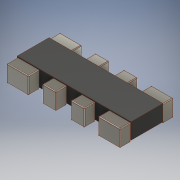
# Autodesk Inventor part: ResistorArray-1632
Saved by Autodesk Inventor 2018 (Build 220112000, 112)
## iProperties
Created: 2018-09-29
Part Number: ResistorArray-1632
Material: Copper
Document SubType Name: Modeling
Designer: Bradley
Density: 8.94 g/cm^3
Appearance: Copper - Satin
Author: Bradley
Autodesk Inventor part; units mm, degrees
ref_plane "YZ Plane" through (0, 0, 0) normal (1, 0, 0) x (0, 1, 0)
ref_plane "XZ Plane" through (0, 0, 0) normal (0, 1, 0) x (-1, 0, 0)
ref_plane "XY Plane" through (0, 0, 0) normal (0, 0, 1) x (1, 0, 0)
sketch "Sketch1" plane through (0, 0, 0) normal (0, 0, 1) x (1, 0, 0)
  line L0 (-1.6, -0.45) -> (1.6, -0.45)
  line L1 (1.6, -0.45) -> (1.6, 0.45)
  line L2 (1.6, 0.45) -> (-1.6, 0.45)
  line L3 (-1.6, 0.45) -> (-1.6, -0.45)
  line L4 (-1.6, -0.45) -> (1.6, 0.45) construction
  line L5 (1.6, -0.45) -> (-1.6, 0.45) construction
  point P0 (0, 0)
  dimension "d0" = 3.2
  dimension "d1" = 0.9
  constraints: 12 end point, 2 midpoint, 2 parallel, 1 horizontal, 1 perpendicular
  measures "d0" distance of L2.end L1.end
  measures "d1" distance of L2.end L0.start
extrude "Extrusion1" add sketch "Sketch1" along normal mid plane 0.45
sketch "Sketch2" plane through (0, 0, 0) normal (0, 0, 1) x (1, 0, 0)
  line L0 (-1.6, -0.45) -> (1.6, -0.45) projected
  line L1 (1.6, -0.45) -> (1.6, 0.45) projected
  line L2 (1.6, 0.45) -> (-1.6, 0.45) projected
  line L3 (-1.6, 0.45) -> (-1.6, -0.45) projected
  line L4 (1.6, 0.45) -> (-1.6, 0.45) projected
  line L5 (-1.59, 0.45) -> (-0.98, 0.45)
  line L6 (-0.98, 0.45) -> (-0.98, 0.75)
  line L7 (-0.98, 0.75) -> (-1.59, 0.75)
  line L8 (-1.59, 0.75) -> (-1.59, 0.45)
  line L9 (1.59, -0.45) -> (0.98, -0.45)
  line L10 (0.98, -0.45) -> (0.98, -0.75)
  line L11 (0.98, -0.75) -> (1.59, -0.75)
  line L12 (1.59, -0.75) -> (1.59, -0.45)
  line L13 (1.59, 0.45) -> (0.98, 0.45)
  line L14 (0.98, 0.45) -> (0.98, 0.75)
  line L15 (0.98, 0.75) -> (1.59, 0.75)
  line L16 (1.59, 0.75) -> (1.59, 0.45)
  line L17 (-0.59, 0.45) -> (-0.21, 0.45)
  line L18 (-0.21, 0.45) -> (-0.21, 0.75)
  line L19 (-0.21, 0.75) -> (-0.59, 0.75)
  line L20 (-0.59, 0.75) -> (-0.59, 0.45)
  line L21 (-1.6, -0.45) -> (1.6, -0.45) projected
  line L22 (-0.59, -0.45) -> (-0.21, -0.45)
  line L23 (-0.21, -0.45) -> (-0.21, -0.75)
  line L24 (-0.21, -0.75) -> (-0.59, -0.75)
  line L25 (-0.59, -0.75) -> (-0.59, -0.45)
  line L26 (0.21, -0.45) -> (0.59, -0.45)
  line L27 (0.59, -0.45) -> (0.59, -0.75)
  line L28 (0.59, -0.75) -> (0.21, -0.75)
  line L29 (0.21, -0.75) -> (0.21, -0.45)
  line L30 (0.59, 0.75) -> (0.21, 0.75)
  line L31 (0.21, 0.75) -> (0.21, 0.45)
  line L32 (0.59, 0.45) -> (0.59, 0.75)
  line L33 (0.21, 0.45) -> (0.59, 0.45)
  line L34 (1.6, -0.45) -> (-1.6, -0.45) projected
  line L35 (-1.59, -0.45) -> (-0.98, -0.45)
  line L36 (-0.98, -0.45) -> (-0.98, -0.75)
  line L37 (-0.98, -0.75) -> (-1.59, -0.75)
  line L38 (-1.59, -0.75) -> (-1.59, -0.45)
  point P0 (0, 0)
  point P1 (0.4, 0.75)
  dimension "d4" = 0.61
  dimension "d5" = 0.38
  dimension "d9" = 0.8
  dimension "d18" = 0.01
  dimension "d19" = 0.01
  dimension "d25" = 0.4
  dimension "d26" = 1.5
  constraints: 64 end point, 12 parallel, 10 collinear, 10 point on line, 7 horizontal, 6 perpendicular, 1 midpoint, 17 other
  measures "d4" distance of L6.end L7.end
  measures "d5" distance of L18.end L19.end
  measures "d9" distance of L22.end L26.end
  measures "d18" distance between parallel lines of L1 L16
  measures "d19" distance between parallel lines of L3 L8
  measures "d25" horizontal distance of point (0, 0) point (0.4, 0.75)
  measures "d26" distance between parallel lines of L37 L7
extrude "Extrusion2" add sketch "Sketch2" along normal blind 0.2 and the other way blind 0.275 contours L0 L36 L37 L38 | L8 L7 L6 L2 | L0 L23 L24 L25 | L20 L19 L18 L2 | L0 L27 L28 L29 | L31 L30 L32 L2 | L0 L12 L11 L10 | L14 L15 L16 L2
fillet "Fillet1" radius 0.02 88 edges at (0.98, 0.45, -0.25) (1.285, 0.45, -0.275) (1.59, 0.45, -0.25) (1.59, 0.6, -0.275) (0.98, 0.6, -0.275) (1.285, 0.75, -0.275) (0.98, 0.6, 0.2) (0.98, 0.75, -0.0375) (1.285, 0.75, 0.2) (1.59, 0.75, -0.0375) (1.59, 0.6, 0.2) (1.285, -0.45, -0.275) (1.59, -0.6, -0.275) (1.285, -0.75, -0.275) (0.98, -0.6, -0.275) (1.59, -0.6, 0.2) (1.59, -0.75, -0.0375) (1.59, -0.45, -0.25) (1.285, -0.75, 0.2) (0.98, -0.75, -0.0375) (0.98, -0.6, 0.2) (0.98, -0.45, -0.25) (0.4, -0.45, -0.275) (0.59, -0.6, -0.275) (0.4, -0.75, -0.275) (0.21, -0.6, -0.275) (0.59, -0.6, 0.2) (0.59, -0.75, -0.0375) (0.59, -0.45, -0.25) (0.4, -0.75, 0.2) (0.21, -0.75, -0.0375) (0.21, -0.6, 0.2) (0.21, -0.45, -0.25) (-0.21, -0.45, -0.25) (-0.4, -0.45, -0.275) (-0.59, -0.45, -0.25) (-0.59, -0.6, -0.275) (-0.21, -0.6, -0.275) (-0.4, -0.75, -0.275) (-0.21, -0.6, 0.2) (-0.21, -0.75, -0.0375) (-0.4, -0.75, 0.2) (-0.59, -0.75, -0.0375) (-0.59, -0.6, 0.2) (-0.4, 0.45, -0.275) (-0.59, 0.6, -0.275) (-0.4, 0.75, -0.275) (-0.21, 0.6, -0.275) (-0.59, 0.6, 0.2) (-0.59, 0.75, -0.0375) (-0.59, 0.45, -0.25) (-0.4, 0.75, 0.2) (-0.21, 0.75, -0.0375) (-0.21, 0.6, 0.2) (-0.21, 0.45, -0.25) (0.4, 0.45, -0.275) (0.21, 0.6, -0.275) (0.4, 0.75, -0.275) (0.59, 0.6, -0.275) (0.21, 0.6, 0.2) (0.21, 0.75, -0.0375) (0.21, 0.45, -0.25) (0.4, 0.75, 0.2) (0.59, 0.75, -0.0375) (0.59, 0.6, 0.2) (0.59, 0.45, -0.25) (-1.285, 0.45, -0.275) (-1.59, 0.6, -0.275) (-1.285, 0.75, -0.275) (-0.98, 0.6, -0.275) (-1.59, 0.6, 0.2) (-1.59, 0.75, -0.0375) (-1.59, 0.45, -0.25) (-1.285, 0.75, 0.2) (-0.98, 0.75, -0.0375) (-0.98, 0.6, 0.2) (-0.98, 0.45, -0.25) (-0.98, -0.45, -0.25) (-1.285, -0.45, -0.275) (-1.59, -0.45, -0.25) (-1.59, -0.6, -0.275) (-0.98, -0.6, -0.275) (-1.285, -0.75, -0.275) (-0.98, -0.6, 0.2) (-0.98, -0.75, -0.0375) (-1.285, -0.75, 0.2) (-1.59, -0.75, -0.0375) (-1.59, -0.6, 0.2)
equation "\"d19\" = d18"
equation "\"d25\" = 0.5 * d9"
body "Solid1"
